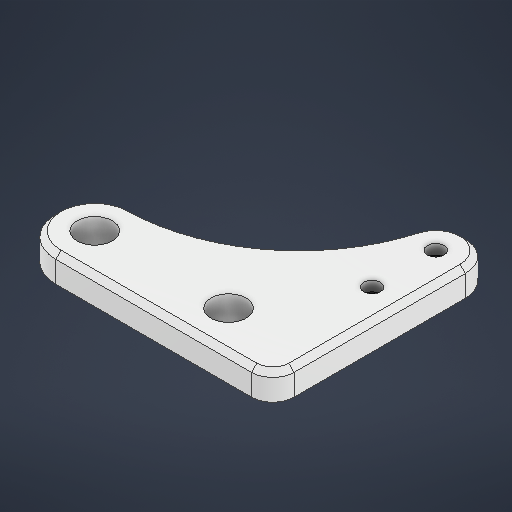
# Autodesk Inventor part: CNC-021-ZAxisLimitSwitchMount
Saved by Autodesk Inventor 2026.2 (Build 302298000, 298)
## iProperties
Created: 2026-06-23
Part Number: CNC-021-ZAxisLimitSwitchMount
Material: ABS Plastic
Document SubType Name: Modeling
Designer: Kenji
Density: 1.06 g/cm^3
Appearance: Smooth - White
Author: Kenji
Autodesk Inventor part; units mm, degrees
ref_plane "YZ Plane" through (0, 0, 0) normal (1, 0, 0) x (0, 1, 0)
ref_plane "XZ Plane" through (0, 0, 0) normal (0, 1, 0) x (-1, 0, 0)
ref_plane "XY Plane" through (0, 0, 0) normal (0, 0, 1) x (1, 0, 0)
sketch "Sketch1" plane through (0, 0, 0) normal (0, 1, 0) x (-1, 0, 0)
  circle A0 centre (0, 0) radius 2.63
  circle A1 centre (20, 0) radius 2.63
  circle A2 centre (-8, -13.4465) radius 1.25
  circle A3 centre (-8, -22.9715) radius 1.25
  circle A4 centre (20, 0) radius 5.805 construction
  circle A5 centre (0, 0) radius 5.805 construction
  circle A6 centre (-8, -13.4465) radius 4.425 construction
  circle A7 centre (-8, -22.9715) radius 4.425 construction
  line L0 (20, 5.805) -> (-9.25, 5.805)
  line L1 (-12.425, 2.63) -> (-12.425, -22.9715)
  line L2 (23.5083, -4.625) -> (-5.3257, -26.497)
  arc A8 (23.5083, -4.625) -> (20, 5.805) centre (20, 0) ccw
  arc A9 (-12.425, -22.9715) -> (-5.3257, -26.497) centre (-8, -22.9715) ccw
  arc A10 (-9.25, 5.805) -> (-12.425, 2.63) centre (-9.25, 2.63) ccw
  point P0 (0, 10)
  dimension "d0" = 5.26
  dimension "d1" = 20
  dimension "d2" = 2.5
  dimension "d3" = 10
  dimension "d4" = 13.4465
  dimension "d5" = 8
  dimension "d6" = 9.525
  dimension "d7" = 3.175
  dimension "d8" = 3.175
  dimension "d9" = 3.175
  constraints: 11 centre point, 10 point on circle, 8 tangent, 6 end point, 5 equal radius, 4 coincident, 2 vertical alignment, 1 horizontal, 1 horizontal alignment, 1 perpendicular
  measures "d0" diameter of A0
  measures "d1" distance of point (0, 0) A1.centre
  measures "d2" diameter of A2
  measures "d3" distance of point (0, 0) point (0, 10)
  measures "d4" vertical distance of A2.centre point (0, 0)
  measures "d5" horizontal distance of A2.centre point (0, 0)
  measures "d6" distance of A3.centre A2.centre
  measures "d7" radial gap between concentric circles of A4 A1
  measures "d8" radial gap between concentric circles of A2 A6
  measures "d9" radius of A10
extrude "Extrusion1" add sketch "Sketch1" along normal blind 4
sketch "Sketch2" plane through (0, 0, 0) normal (0, -1, 0) x (1, 0, 0)
  circle A0 centre (8, -13.4465) radius 1.25 projected
  circle A1 centre (8, -22.9715) radius 1.25 projected
  circle A2 centre (8, -13.4465) radius 2
  circle A3 centre (8, -22.9715) radius 2
  point P0 (0, 0)
  dimension "d12" = 4
  constraints: 2 centre point, 2 coincident, 1 equal radius
  measures "d12" diameter of A2
extrude "Extrusion2" cut sketch "Sketch2" against normal blind 2.5
sketch "Sketch3" plane through (0, 4, 0) normal (0, 1, 0) x (1, 0, 0)
  circle A0 centre (-20, 0) radius 2.63 projected
  circle A1 centre (8, 22.9715) radius 1.25 projected
  circle A2 centre (-20, 0) radius 5.805 construction
  circle A3 centre (8, 22.9715) radius 4.425 construction
  arc A4 (-23.5083, 4.625) -> (-20, -5.805) centre (-20, 0) ccw projected
  arc A5 (12.425, 22.9715) -> (5.3257, 26.497) centre (8, 22.9715) ccw projected
  circle A6 centre (0, 0) radius 5.805 construction
  circle A7 centre (8, 13.4465) radius 1.25 construction
  circle A8 centre (8, 13.4465) radius 4.425 construction
  arc A9 (-20.1243, 5.8037) -> (3.7466, 24.192) centre (-20.6681, 31.1978) ccw
  arc A10 (-20.1243, 5.8037) -> (-23.5083, 4.625) centre (-20, 0) ccw
  arc A11 (5.3257, 26.497) -> (3.7466, 24.192) centre (8, 22.9715) ccw
  line L0 (5.3257, 26.497) -> (-23.5083, 4.625) projected
  dimension "d15" = 25.4
  constraints: 6 point on circle, 5 centre point, 2 coincident, 1 equal radius, 13 other
  measures "d15" radius of A9
extrude "Extrusion3" cut sketch "Sketch3" against normal through all contours A10 L0 A11 A9
chamfer "Chamfer1" distance 0.7937 angle 45 6 edges at (12.425, 4, -10.1707) (8.6163, 4, -27.3534) (-5.1676, 4, -11.0758) (-25.8047, 4, 0.0621) (-5.375, 4, 5.805) (11.4951, 4, 4.8751)
body "Solid1"
